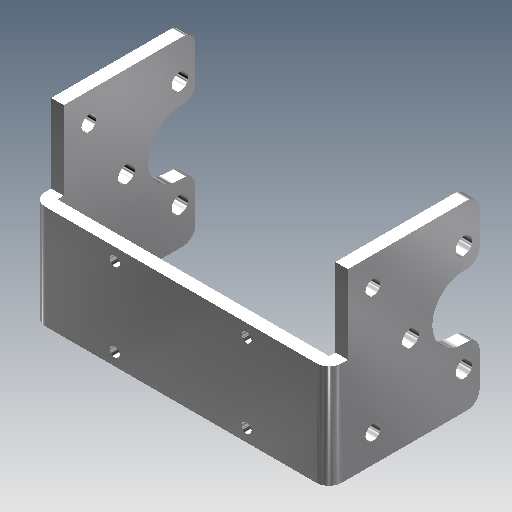
# Autodesk Inventor part: 頭_メインフレーム_1_2
Saved by Autodesk Inventor 2017.3 (Build 213256000, 256)
## iProperties
Created: 2016-05-10
Part Number: 頭_メインフレーム_1_2
Material: アルミニウム 5052
Document SubType Name: シート メタル
Designer: hiroaki
Density: 2.68 g/cm^3
Appearance: アルミニウム - フラット
Sheet Metal Rule: Default_mm
Mass: 8.3517 g
Surface Area: 40.402 cm^2
Volume: 3.11631 cm^3
Flat Pattern Width: 2.9 cm
Flat Pattern Length: 9.00647 cm
Flat Pattern Area: 26.1188 cm^2
Sheet Metal Width: 29.000 mm
Sheet Metal Length: 90.065 mm
Sheet Metal Area: 2611.877 mm^2
Author: hiroaki
Autodesk Inventor part; units mm, degrees
ref_plane "YZ Plane" through (0, 0, 0) normal (1, 0, 0) x (0, 1, 0)
ref_plane "XZ Plane" through (0, 0, 0) normal (0, 1, 0) x (-1, 0, 0)
ref_plane "XY Plane" through (0, 0, 0) normal (0, 0, 1) x (1, 0, 0)
sketch "スケッチ1" plane through (0, 0, 0) normal (0, 0, 1) x (1, 0, 0)
  line L0 (-21.65, -14.5) -> (21.65, -14.5)
  line L1 (21.65, -14.5) -> (21.65, 14.5)
  line L2 (21.65, 14.5) -> (-21.65, 14.5)
  line L3 (-21.65, 14.5) -> (-21.65, -14.5)
  line L4 (-21.65, -14.5) -> (21.65, 14.5) construction
  line L5 (21.65, -14.5) -> (-21.65, 14.5) construction
  line L6 (-10.5, 0) -> (10.5, 0) construction
  line L7 (10.5, 0) -> (10.5, -12.5) construction
  line L8 (10.5, -12.5) -> (-10.5, -12.5) construction
  line L9 (-10.5, -12.5) -> (-10.5, 0) construction
  circle A0 centre (-10.5, 0) radius 0.8
  circle A1 centre (10.5, 0) radius 0.8
  circle A2 centre (10.5, -12.5) radius 0.8
  circle A3 centre (-10.5, -12.5) radius 0.8
  point P0 (0, 0)
  point P1 (0, 0)
  point P2 (0, 0)
  point P3 (0, 0)
  dimension "d0" = 21
  dimension "d1" = 12.5
  dimension "d2" = 1.6
  dimension "d3" = 2
  dimension "d4" = 43.3
  constraints: 20 end point, 6 midpoint, 5 coincident, 4 centre point, 4 parallel, 3 equal radius, 2 horizontal, 2 perpendicular
  measures "d0" distance of L6.start L6.end
  measures "d1" distance of L6.end L7.end
  measures "d2" diameter of A0
  measures "d3" distance between parallel lines of L0 L8
  measures "d4" distance of L1.end L2.end
extrude "押し出し1" add sketch "スケッチ1" along normal blind 2
sketch "スケッチ2" plane through (21.6501, -14.5, -0.0001) normal (1, 0, 0) x (0, 1, 0)
  line L0 (29, 0) -> (0, 0)
  line L1 (0, 0) -> (0, -21.9999)
  line L2 (0, -21.9999) -> (29, -21.9999)
  line L3 (29, -21.9999) -> (29, 0)
  constraints: 6 end point, 1 horizontal, 1 perpendicular, 1 vertical
edge flange "フランジ1" height 22 angle 90 thickness 2 bend radius 0.0001 thickness toward (1, 0, 0) relief straight relief width 2 relief depth 1 edges at (21.65, 0, 0) wall of the first edge with corners at (21.6501, 14.5, -0.0001) (21.6501, -14.5, -0.0001) (21.6501, -14.5, -22) (21.6501, 14.5, -22)
bend "曲げ1"
corner "コーナー1"
sketch "スケッチ3" plane through (23.6501, -14.5, -22) normal (1, 0, 0) x (0, 0, -1)
  line L0 (-21.9999, 29) -> (-21.9999, 0) projected
  circle A0 centre (-2.4999, 14.5) radius 11 construction
  line L1 (-14.4999, 3.917) -> (-14.4999, 25.083) construction
  arc A1 (-14.4999, 3.917) -> (-12.9902, 2.4188) centre (-2.4999, 14.5) ccw construction
  circle A2 centre (-2.4999, 14.5) radius 17.5 construction
  circle A3 centre (-2.4999, 14.5) radius 19.5 construction
  circle A4 centre (-2.4999, 14.5) radius 5.05
  circle A5 centre (-10.9999, 14.5) radius 1.35
  circle A6 centre (-2.4999, 6) radius 1.35
  circle A7 centre (6.0001, 14.5) radius 1.35
  circle A8 centre (-2.4999, 23) radius 1.35
  circle A9 centre (-2.4999, 6) radius 2.5 construction
  line L2 (0.0001, -5.061) -> (0.0001, 35.0453) construction
  circle A10 centre (-17, 4.5) radius 1.2
  circle A11 centre (-17, 24.5) radius 1.2
  line L3 (-24, 0) -> (-24, 29) projected
  point P0 (-22, 14.5)
  point P1 (-21.9999, 14.5)
  point P2 (-14.4999, 14.5)
  dimension "d17" = 22
  dimension "d18" = 12
  dimension "d19" = 16
  dimension "d20" = 35
  dimension "d21" = 2
  dimension "d22" = 10.1
  dimension "d23" = 2.7
  dimension "d24" = 8.5
  dimension "d27" = 360
  dimension "d35" = 2.4
  dimension "d36" = 20
  dimension "d37" = 10
  dimension "d38" = 7
  constraints: 12 centre point, 4 coincident, 4 end point, 3 horizontal alignment, 3 tangent, 2 midpoint, 2 point on circle, 2 vertical, 1 equal radius, 1 vertical alignment, 9 other
  measures "d17" diameter of A0
  measures "d18" distance from line of A0.centre L1
  measures "d19" radius of A1
  measures "d20" diameter of A2
  measures "d21" radial gap between concentric circles of A3 A2
  measures "d22" diameter of A4
  measures "d23" diameter of A5
  measures "d24" distance of A0.centre A5.centre
  measures "d35" diameter of A10
  measures "d36" distance of A11.centre A10.centre
  measures "d37" vertical distance of point (-14.5, 14.5) A11.centre
  measures "d38" distance from line of L3 A10.centre
extrude "押し出し2" cut sketch "スケッチ3" against normal blind 2 contours A4 | A5 | A6 | A8 | A10 | A11
fillet "フィレット1" radius 2 4 edges at (22.6501, -4.3878, -22) (22.6501, 4.3878, -22) (22.6501, 14.5, -22) (22.6501, -14.5, -22)
mirror "ミラー1" about plane through (0, 0, 0) normal (1, 0, 0) of "フランジ1", "押し出し2", "フィレット1"
sketch "スケッチ4" plane through (0, 0, 2) normal (0, 0, 1) x (1, 0, 0)
  circle A0 centre (10.5, -12.5) radius 0.8 projected
  circle A1 centre (10.5, 0) radius 0.8 projected
  line L0 (-21.65, -14.5) -> (21.65, -14.5) projected
  line L1 (32.6032, 2) -> (-36.1158, 2)
  line L2 (-36.1158, 2) -> (-36.1158, 15.5279)
  line L3 (-36.1158, 15.5279) -> (32.6032, 15.5279)
  line L4 (32.6032, 15.5279) -> (32.6032, 2)
  circle A2 centre (10.5, -12.5) radius 2 construction
  circle A3 centre (10.5, 0) radius 2 construction
  line L5 (21.65, -14.5) -> (21.65, 14.5) projected
  line L6 (-21.65, 14.5) -> (-21.65, -14.5) projected
  line L7 (17.65, -10) -> (-17.65, -10)
  line L8 (-17.65, -10) -> (-17.65, -2.5)
  line L9 (-17.65, -2.5) -> (17.65, -2.5)
  line L10 (17.65, -2.5) -> (17.65, -10)
  point P0 (0, 0)
  dimension "d39" = 2.5
  dimension "d40" = 2.5
  dimension "d41" = 4
  dimension "d42" = 4
  constraints: 16 end point, 4 parallel, 2 centre point, 2 coincident, 2 horizontal, 2 perpendicular, 2 tangent, 1 equal radius
  measures "d39" distance from line of A0.centre L7
  measures "d40" distance from line of A1.centre L9
  measures "d41" distance between parallel lines of L5 L10
  measures "d42" distance between parallel lines of L6 L8
extrude "押し出し3" cut sketch "スケッチ4" against normal blind 3 contours L1 L2 L3 L4
equation "\"d37\" = 0.5 * d36"
equation "\"d40\" = d39"
equation "\"d42\" = d41"
equation "\"d7\" = BendReliefWidth"
equation "\"d8\" = BendReliefDepth"
equation "\"d9\" = MinimumRemnant"
equation "\"d10\" = BendRadius"
equation "\"d14\" = CornerReliefSize"
equation "\"d15\" = GapSize"
equation "\"d16\" = JacobiRadiusSize"
equation "\"BendRadius\" = Thickness"
equation "\"BendReliefWidth\" = Thickness"
equation "\"BendReliefDepth\" = 0.5 * Thickness"
equation "\"CornerReliefSize\" = 4 * Thickness"
equation "\"MinimumRemnant\" = 2 * Thickness"
equation "\"TransitionRadius\" = BendRadius"
equation "\"JacobiRadiusSize\" = BendRadius"
equation "\"GapSize\" = Thickness"
equation "\"Thickness\" = 2"
